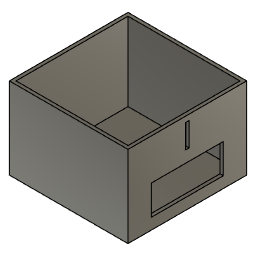
pechat v1 (Autodesk Fusion 360 design; units mm, degrees)
Autodesk Fusion 360 part; units mm, degrees
sketch "Sketch1" plane through (0, 0, 0) normal (0, 0, 1) x (1, 0, 0)
  line L0 (-80, 80) -> (80, 80)
  line L1 (80, 80) -> (80, -80)
  line L2 (80, -80) -> (-80, -80)
  line L3 (-80, -80) -> (-80, 80)
  line L4 (-80, 80) -> (80, -80) construction
  line L5 (80, 80) -> (-80, -80) construction
  dimension "d1" = 160
  dimension "d3" = 160
  constraint horizontal L0
  constraint perpendicular L0 L1
  constraint parallel L0 L2
  constraint parallel L1 L3
  constraint coincident L4 origin
  constraint coincident L5 origin
  measures "d1" distance of L1.end L2.end
  measures "d3" distance of L0.start L2.end
extrude "Extrude1" add sketch "Sketch1" along normal blind 110
sketch "Sketch3" plane through (0, 0, 110) normal (0, 0, 1) x (-1, 0, 0)
  line L0 (80, 80) -> (-80, 80)
  line L1 (-80, 80) -> (-80, -80)
  line L2 (-80, -80) -> (80, -80)
  line L3 (80, -80) -> (80, 80)
  line L4 (75.5, -75.5) -> (-75.5, -75.5)
  line L5 (-75.5, -75.5) -> (-75.5, 75.5)
  line L6 (-75.5, 75.5) -> (75.5, 75.5)
  line L7 (75.5, 75.5) -> (75.5, -75.5)
  line L8 (75.5, -75.5) -> (-75.5, 75.5) construction
  line L9 (-75.5, -75.5) -> (75.5, 75.5) construction
  dimension "d7" = 151
  dimension "d8" = 151
  constraint horizontal L4
  constraint perpendicular L4 L5
  constraint parallel L4 L6
  constraint parallel L5 L7
  constraint coincident L8 origin
  constraint coincident L9 origin
  measures "d7" distance of L5.end L6.end
  measures "d8" distance of L4.end L5.end
extrude "Extrude2" cut sketch "Sketch3" against normal blind 105.5 contours L4 L5 L6 L7
sketch "Sketch4" plane through (80, 0, 0) normal (1, 0, 0) x (0, 1, 0)
  line L0 (-80, 0) -> (80, 0)
  line L1 (80, 0) -> (80, 110)
  line L2 (80, 110) -> (-80, 110)
  line L3 (-80, 110) -> (-80, 0)
  line L4 (2.5, 70.5) -> (-2.5, 70.5)
  line L5 (-2.5, 70.5) -> (-2.5, 102.5)
  line L6 (-2.5, 102.5) -> (2.5, 102.5)
  line L7 (2.5, 102.5) -> (2.5, 70.5)
  line L8 (2.5, 70.5) -> (-2.5, 102.5) construction
  line L9 (-2.5, 70.5) -> (2.5, 102.5) construction
  point P0 (0, 86.5)
  dimension "d11" = 7.5
  dimension "d12" = 32
  dimension "d13" = 5
  dimension "d14" = 77.5
  constraint horizontal L4
  constraint perpendicular L4 L5
  constraint parallel L4 L6
  constraint parallel L5 L7
  constraint coincident L8 P0
  constraint coincident L9 P0
  measures "d11" distance of L2 L6
  measures "d12" distance of L4.start L6.end
  measures "d13" distance of L4.start L4.end
  measures "d14" distance of L1 L7
extrude "Extrude3" cut sketch "Sketch4" against normal blind 5 contours L4 L5 L6 L7
sketch "Sketch5" plane through (80, 0, 0) normal (1, 0, 0) x (0, 1, 0)
  line L0 (-2.5, 70.5) -> (-2.5, 102.5)
  line L1 (-2.5, 102.5) -> (2.5, 102.5)
  line L2 (2.5, 102.5) -> (2.5, 70.5)
  line L3 (2.5, 70.5) -> (-2.5, 70.5)
  line L4 (-80, 0) -> (80, 0)
  line L5 (80, 0) -> (80, 110)
  line L6 (80, 110) -> (-80, 110)
  line L7 (-80, 110) -> (-80, 0)
  line L8 (48.5, 55) -> (-48.5, 55)
  line L9 (-48.5, 55) -> (-48.5, 15)
  line L10 (-48.5, 15) -> (48.5, 15)
  line L11 (48.5, 15) -> (48.5, 55)
  line L12 (48.5, 55) -> (-48.5, 15) construction
  line L13 (-48.5, 55) -> (48.5, 15) construction
  point P0 (0, 35)
  dimension "d17" = 97
  dimension "d18" = 31.5
  dimension "d19" = 40
  dimension "d20" = 15
  constraint horizontal L8
  constraint perpendicular L8 L9
  constraint parallel L8 L10
  constraint parallel L9 L11
  constraint coincident L12 P0
  constraint coincident L13 P0
  measures "d17" distance of L8.start L8.end
  measures "d18" distance of L5 L11
  measures "d19" distance of L8.end L9.end
  measures "d20" distance of L4 L10
extrude "Extrude4" cut sketch "Sketch5" against normal blind 5 contours L8 L9 L10 L11
equation "d1 = Cube_size"
equation "d3 = Cube_size"
equation "Cube_size = 160 mm"
equation "d5 = Cube_size / 16 * 11"
equation "d7 = Cube_size - Cube_size * 0.05625"
equation "d8 = Cube_size - Cube_size * 0.05625"
equation "d9 = 0.6875 * Cube_size * 0.0409090909090909 - 0.6875 * Cube_size"
equation "d11 = 0.6875 * Cube_size * 0.0681818181818182"
equation "d12 = 0.6875 * Cube_size * 0.2909090909090909"
equation "d13 = 0.0454545454545455 * 0.6875 * Cube_size"
equation "d14 = ( Cube_size - 0.0454545454545455 * 0.6875 * Cube_size ) / 2"
equation "d15 = -Cube_size * 0.03125"
equation "d17 = Cube_size * 0.60625"
equation "d18 = Cube_size * 0.196875"
equation "d19 = 0.25 * Cube_size"
equation "d20 = Cube_size * 0.09375"
equation "d21 = -Cube_size * 0.03125"
